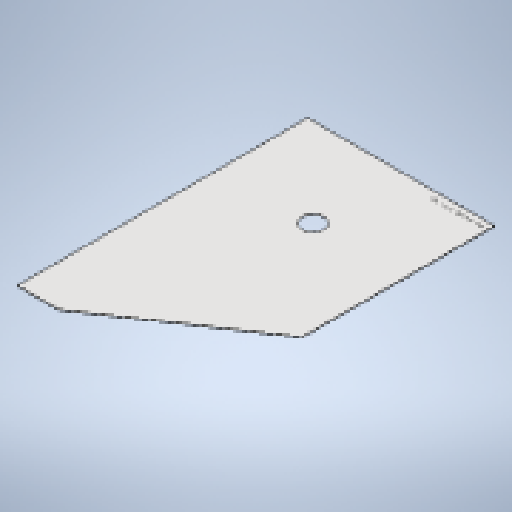
# Autodesk Inventor part: TRM 015 left board main
Saved by Autodesk Inventor 2025 (Build 290162010, 162A)
## iProperties
Created: 2024-08-07
Part Number: TRM 015 left board main
Material: AISI 304
Document SubType Name: Sheet Metal
Designer: pokla
Density: 8.02768 g/cm^3
Flat Pattern Width: 67.6462 cm
Flat Pattern Length: 105 cm
Flat Pattern Area: 7102.85 cm^2
Sheet Metal Rule: AISI304 2mm Die16
Sheet Metal Width: 676,462 mm
Sheet Metal Length: 1050,000 mm
Sheet Metal Area: 710284,791 mm^2
Appearance: Default
Stock Number: ТРМ 015 левый борт основное
Author: pokla
Autodesk Inventor part; units mm, degrees
ref_plane "YZ Plane" through (0, 0, 0) normal (1, 0, 0) x (0, 1, 0)
ref_plane "XZ Plane" through (0, 0, 0) normal (0, 1, 0) x (-1, 0, 0)
ref_plane "XY Plane" through (0, 0, 0) normal (0, 0, 1) x (1, 0, 0)
sketch "Sketch1" plane through (0, 0, 0) normal (0, 0, 1) x (1, 0, 0)
  line L0 (-339.5757, -526.8077) -> (336.886, -526.8077)
  line L1 (336.886, -526.8077) -> (336.886, 523.1923)
  line L2 (336.886, 523.1923) -> (-339.5757, 523.1923)
  line L3 (-339.5757, 523.1923) -> (-339.5757, -526.8077)
  line L4 (-189.5757, -526.8077) -> (336.886, -173)
  circle A0 centre (0, 203.1923) radius 40
  line L5 (336.886, -173) -> (120.3666, -173)
  line L6 (120.3666, -173) -> (120.3666, -318.5115)
  point P0 (0, 0)
  dimension "d1" = 1050
  dimension "d13" = 150
  dimension "d14" = 80
  dimension "d15" = 320
  measures "d1" distance of L1.end L0.end
  measures "d13" distance of L4.start L0.start
  measures "d14" diameter of A0
  measures "d15" distance from line of A0.centre L2
extrude "Plate1" add sketch "Sketch1" along normal blind 2 contours L3 L2 L1 L5 L6 L4 L0 | L6 L5 L4
sketch "Sketch2" plane through (0, 0, 0) normal (0, 0, -1) x (-1, 0, 0)
  line L0 (-316.886, 503.1923) -> (-116.886, 503.1923) construction
  line L1 (-116.886, 503.1923) -> (-116.886, 483.1923) construction
  line L2 (-116.886, 483.1923) -> (-316.886, 483.1923) construction
  line L3 (-316.886, 483.1923) -> (-316.886, 503.1923) construction
  line L4 (-336.886, 523.1923) -> (339.5757, 523.1923) projected
  line L5 (-336.886, -173) -> (-336.886, 523.1923) projected
  point P0 (0, 0)
  point P1 (-48, 100)
  point P2 (339.5757, 523.1923)
  point P3 (-251, -525)
  point P4 (-50, 98)
  dimension "d6" = 200
  dimension "d9" = 20
  dimension "d10" = 20
  dimension "d11" = 20
  constraints: 4 other
  measures "d6" distance of L0.start L0.end
  measures "d9" distance of L0.end L1.end
  measures "d11" length of L3
mark "Mark1"
equation "\"d2\" = Thickness"
equation "\"BendReliefWidth\" = Thickness"
equation "\"BendReliefDepth\" = 0.5 * Thickness"
equation "\"CornerReliefSize\" = 4 * Thickness"
equation "\"MinimumRemnant\" = 2 * Thickness"
equation "\"TransitionRadius\" = BendRadius"
equation "\"JacobiRadiusSize\" = BendRadius"
equation "\"GapSize\" = Thickness"
equation "\"Thickness\" = 2"
equation "\"BendRadius\" = 2.75"
body "Solid1"
